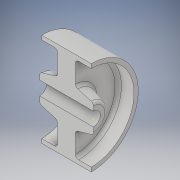
# Autodesk Inventor part: 練習二
Saved by Autodesk Inventor 2017 (Build 210142000, 142)
## iProperties
Part Number: 練習二
Material: 一般
Document SubType Name: Modeling
Designer: user
Density: 1 g/cm^3
Appearance: 預設
Author: user
Autodesk Inventor part; units mm, degrees
ref_plane "YZ Plane" through (0, 0, 0) normal (1, 0, 0) x (0, 1, 0)
ref_plane "XZ Plane" through (0, 0, 0) normal (0, 1, 0) x (-1, 0, 0)
ref_plane "XY Plane" through (0, 0, 0) normal (0, 0, 1) x (1, 0, 0)
sketch "草圖1" plane through (0, 0, 0) normal (0, 0, 1) x (1, 0, 0)
  line L0 (0, 0) -> (0, 13)
  line L1 (0, 13) -> (14.8465, 17.3666)
  line L2 (17, 20.2447) -> (17, 37.5)
  line L3 (14, 40.5) -> (2, 40.5)
  line L4 (2, 44.5) -> (49, 44.5)
  line L5 (49, 40.5) -> (37, 40.5)
  line L6 (34, 37.5) -> (34, 20.2447)
  line L7 (36.1535, 17.3666) -> (51, 13)
  line L8 (51, 13) -> (51, 0)
  line L9 (51, 0) -> (0, 0)
  line L10 (2, 40.5) -> (2, 44.5)
  line L11 (49, 40.5) -> (49, 44.5)
  line L12 (25.5, 0) -> (25.5, 70.2145)
  arc A0 (14.8465, 17.3666) -> (17, 20.2447) centre (14, 20.2447) ccw
  arc A1 (34, 20.2447) -> (36.1535, 17.3666) centre (37, 20.2447) ccw
  arc A2 (17, 37.5) -> (14, 40.5) centre (14, 37.5) ccw
  arc A3 (37, 40.5) -> (34, 37.5) centre (37, 37.5) ccw
  point P0 (17, 18)
  point P1 (17, 40.5)
  point P2 (34, 40.5)
  point P3 (34, 18)
  dimension "d0" = 51
  dimension "d1" = 47
  dimension "d2" = 17
  dimension "d3" = 18
  dimension "d4" = 4
  dimension "d5" = 40.5
  dimension "d6" = 15
  dimension "d7" = 18
  dimension "d8" = 13
  dimension "d9" = 13
  dimension "d10" = 3
  constraints: 30 end point, 10 point on line, 8 point on circle, 8 tangent, 5 vertical, 4 centre point, 3 equal radius, 3 perpendicular, 1 horizontal, 1 midpoint, 1 other
  measures "d0" distance between parallel lines of L8 L0
  measures "d1" distance of L4.start L4.end
  measures "d2" distance between parallel lines of L2 L6
  measures "d3" distance from line of point (17, 18) L9
  measures "d4" distance between parallel lines of L5 L4
  measures "d5" distance between parallel lines of L9 L5
  measures "d6" distance of point (17, 40.5) L3.end
  measures "d7" distance from line of point (34, 18) L9
  measures "d8" distance of L7.end L8.end
  measures "d9" distance of L0.start L0.end
  measures "d10" radius of A0
revolve "迴轉1" add sketch "草圖1" angle 180 about axis through (51, 0, 0) along (-1, 0, 0)
sketch "草圖2" plane through (51, 0, 0) normal (1, 0, 0) x (0, 0, -1)
  circle A0 centre (0, 0) radius 6.5
  dimension "d13" = 13
  constraints: 1 centre point, 1 coincident
  measures "d13" diameter of A0
extrude "擠出1" cut sketch "草圖2" against normal up to next
fillet "圓角1" radius 3 2 edges at (51, 0, -13) (0, 0, -13)
sketch "草圖3" plane through (51, 0, 0) normal (1, 0, 0) x (0, 0, -1)
  point P0 (0, 0)
